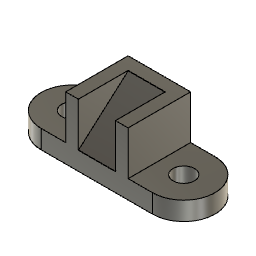
A2 v1 (Autodesk Fusion 360 design; units mm, degrees)
Autodesk Fusion 360 part; units mm, degrees
sketch "Sketch1" plane through (0, 0, 0) normal (0, 0, 1) x (1, 0, 0)
  line L0 (57, -32) -> (-57, -32)
  line L1 (-57, 32) -> (57, 32)
  circle A0 centre (-57, 0) radius 11
  circle A1 centre (57, 0) radius 11
  arc A2 (57, -32) -> (57, 32) centre (57, 0) ccw
  arc A3 (-57, 32) -> (-57, -32) centre (-57, 0) ccw
  dimension "d1" = 114
  dimension "d2" = 64
  dimension "d7" = 22
  dimension "d8" = 22
  constraint horizontal L0
  constraint parallel L0 L1
  measures "d1" distance of L1.start L1.end
  measures "d2" distance of L0.end L1.start
  measures "d7" diameter of A0
  measures "d8" diameter of A1
extrude "Extrude1" add sketch "Sketch1" along normal blind 19 makes body 1
sketch "Sketch2" plane through (0, 0, 19) normal (0, 0, 1) x (-1, 0, 0)
  circle A0 centre (57, 0) radius 11
  circle A1 centre (-57, 0) radius 11
  arc A2 (-57, 32) -> (-57, -32) centre (-57, 0) ccw
  line L0 (-57, -32) -> (57, -32)
  arc A3 (57, -32) -> (57, 32) centre (57, 0) ccw
  line L1 (57, 32) -> (-57, 32)
  line L2 (32, 32) -> (32, -32)
  line L3 (32, -32) -> (-32, -32)
  line L4 (-32, -32) -> (-32, 32)
  line L5 (-32, 32) -> (-19, 32)
  line L6 (-19, 32) -> (-19, -19)
  line L7 (-19, -19) -> (19, -19)
  line L8 (19, -19) -> (19, 32)
  line L9 (19, 32) -> (32, 32)
  dimension "d11" = 64
  dimension "d12" = 38
  dimension "d14" = 25
  dimension "d15" = 13
  dimension "d16" = 51
  constraint coincident L1 L2.start
  constraint coincident L0 L2.end
  constraint perpendicular L0 L2
  constraint coincident L0 L3.end
  constraint coincident L1 L4.end
  constraint perpendicular L1 L4
  constraint coincident L1 L5.end
  constraint perpendicular L5 L6
  constraint perpendicular L6 L7
  constraint coincident L1 L8.end
  constraint perpendicular L1 L8
  measures "d11" distance of L2.end L3.end
  measures "d12" distance of L6.end L7.end
  measures "d14" distance of A2.start L4.end
  measures "d15" distance of L4.end L5.end
  measures "d16" distance of L7.end L8.end
extrude "Extrude2" add sketch "Sketch2" along normal blind 45 contours L0 L1 L2 L3 L4 L5 L6 L7 L8 L9 bodies 1
sketch "Sketch3" plane through (0, 0, 0) normal (1, 0, 0) x (0, 1, 0)
  line L0 (18.725, 63.9438, 0.3122) -> (18.725, 18.9438, 0.3122)
  line L1 (18.725, 18.9438, 0.3122) -> (-32.275, 18.9438, 0.3122)
  line L2 (-32.275, 18.9438, 0.3122) -> (18.725, 63.9438, 0.3122)
  dimension "d19" = 45
  dimension "d20" = 51
extrude "Extrude3" add sketch "Sketch3" along normal mid plane 38 separate body contours L0 L1 L2 in plane through (0.3122, 0, 0) normal (1, 0, 0) makes body 2
combine "Combine1" operation add target body 1 tool bodies 2
equation "d17 = 64 mm - 19 mm"
equation "d19 = 64 mm - 19 mm"
